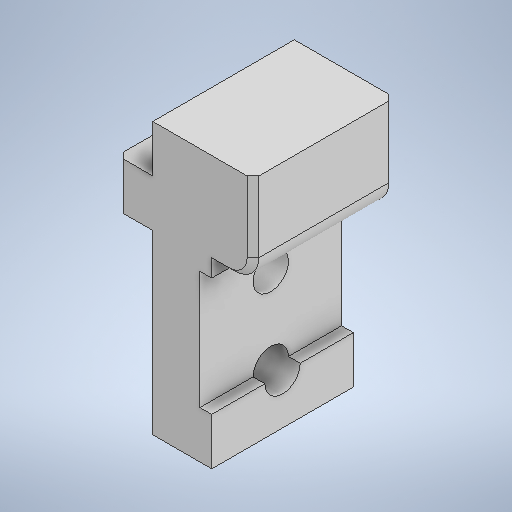
# Autodesk Inventor part: connector
Saved by Autodesk Inventor 2025 (Build 290162000, 162)
## iProperties
Created: 2024-09-26
Part Number: connector
Material: Generic
Document SubType Name: Modeling
Designer: DMIADX
Density: 1 g/cm^3
Appearance: Default
Author: DMIADX
Autodesk Inventor part; units mm, degrees
ref_plane "YZ Plane" through (0, 0, 0) normal (1, 0, 0) x (0, 1, 0)
ref_plane "XZ Plane" through (0, 0, 0) normal (0, 1, 0) x (-1, 0, 0)
ref_plane "XY Plane" through (0, 0, 0) normal (0, 0, 1) x (1, 0, 0)
sketch "Sketch1" plane through (0, 0, 0) normal (0, 0, 1) x (1, 0, 0)
  line L0 (0, 0) -> (0, 4)
  line L1 (0, 4) -> (-1, 4)
  line L2 (-1, 4) -> (-1, 14)
  line L3 (-1, 14) -> (0, 14)
  line L4 (0, 14) -> (0, 15)
  line L5 (0, 15) -> (1.5, 15)
  line L6 (3.5, 17) -> (3.5, 23)
  line L7 (3.5, 23) -> (-5, 23)
  line L8 (-5, 23) -> (-5, 19)
  line L9 (-5, 19) -> (-8, 19)
  line L10 (-8, 19) -> (-8, 15)
  line L11 (-8, 15) -> (-5, 15)
  line L12 (-5, 15) -> (-5, 0)
  line L13 (-5, 0) -> (0, 0)
  arc A0 (1.5, 15) -> (3.5, 17) centre (1.5, 17) ccw
  point P0 (0.75, 15)
  point P1 (-0.5, 4)
  point P2 (0, 2)
  point P3 (-6.5, 15)
  point P4 (-6.5, 19)
  point P5 (-5, 21)
  dimension "d3" = 4
  dimension "d4" = 14
  dimension "d6" = 1
  dimension "d7" = 1
  dimension "d8" = 5
  dimension "d9" = 8
  dimension "d10" = 3
  dimension "d12" = 0
  dimension "d13" = 4
  dimension "d14" = 2
  dimension "d15" = 8.5
  dimension "d16" = 5
  constraints: 28 end point, 12 perpendicular, 6 midpoint, 2 point on circle, 2 point on line, 2 tangent, 1 centre point, 1 vertical
  measures "d3" distance from line of L13 point (-0.5, 4)
  measures "d4" distance from line of L3.end L13
  measures "d6" distance between parallel lines of L3 L5
  measures "d7" distance from line of point (0, 2) L2
  measures "d8" distance between parallel lines of L0 L12
  measures "d9" distance between parallel lines of L5 L7
  measures "d10" distance between parallel lines of L10 L8
  measures "d12" distance between parallel lines of L11 L5
  measures "d13" distance of point (-6.5, 15) point (-6.5, 19)
  measures "d14" radius of A0
  measures "d15" distance from line of L6 point (-5, 21)
  measures "d16" horizontal distance of point (0, 2) point (-5, 21)
extrude "Extrusion1" add sketch "Sketch1" along normal mid plane 12
chamfer "Chamfer1" distance 0.5 angle 45 8 edges at (3.5, 20, 6) (2.9142, 15.5858, 6) (0.75, 15, 6) (-8, 17, 6) (3.5, 20, -6) (2.9142, 15.5858, -6) (0.75, 15, -6) (-8, 17, -6)
sketch "Sketch2" plane through (0, 0, 0) normal (1, 0, 0) x (0, 1, 0)
  circle A0 centre (4, 0) radius 1.5
  circle A1 centre (11, 0) radius 1.5
  line L0 (14, -6) -> (14, 6) projected
  line L1 (0, -6) -> (0, 6) projected
  point P0 (0, 0)
  point P1 (0, 0)
  point P2 (0, 0)
  dimension "d22" = 3
  dimension "d23" = 3
  dimension "d24" = 7
  dimension "d25" = 3
  dimension "d26" = 0
  dimension "d27" = 0
  constraints: 2 centre point, 2 midpoint
  measures "d22" diameter of A0
  measures "d23" diameter of A1
  measures "d24" distance of A0.centre A1.centre
  measures "d25" distance from line of L0 A1.centre
  measures "d26" vertical distance of point (0, 0) A1.centre
  measures "d27" vertical distance of point (0, 0) A0.centre
extrude "Extrusion2" cut sketch "Sketch2" against normal through all
body "Solid1"
